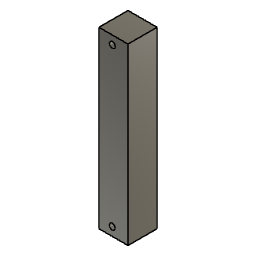
连接柱 v1 (Autodesk Fusion 360 design; units mm, degrees)
Autodesk Fusion 360 part; units mm, degrees
sketch "草图1" plane through (0, 0, 0) normal (0, 0, 1) x (1, 0, 0)
  line L0 (0, 15) -> (5, 15)
  line L1 (5, 15) -> (5, 10)
  line L2 (5, 10) -> (0, 10)
  line L3 (0, 10) -> (0, 15)
  dimension "d1" = 5
  constraint horizontal L0
  constraint vertical L1
  constraint horizontal L2
  constraint vertical L3
  measures "d1" distance of L0.start L0.end
extrude "拉伸1" add sketch "草图1" along normal blind 20
hole "孔1" at (2.293, 10, 1.4617) direction (0, 1, 0) diameter 1 depth 6 tip angle 118
extrude "拉伸2" add 1 faces at (1.6667, 13.3333, 20) along direction (0, 0, 1) blind 10
hole "孔2" at (2.3137, 15, 28.5345) direction (0, -1, 0) diameter 1 depth 6 tip angle 118
